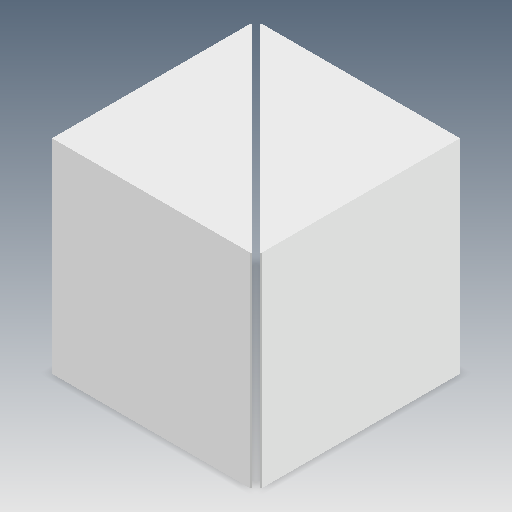
# Autodesk Inventor part: Beamsplittertransparent
Saved by Autodesk Inventor 2026 (Build 300175050, 175E)
## iProperties
Created: 2025-08-02
Part Number: Beamsplittertransparent
Material: Generic
Document SubType Name: Modeling
Designer: aman0
Density: 1 g/cm^3
Appearance: Default
Author: aman0
Autodesk Inventor part; units mm, degrees
ref_plane "YZ Plane" through (0, 0, 0) normal (1, 0, 0) x (0, 1, 0)
ref_plane "XZ Plane" through (0, 0, 0) normal (0, 1, 0) x (-1, 0, 0)
ref_plane "XY Plane" through (0, 0, 0) normal (0, 0, 1) x (1, 0, 0)
sketch "Sketch1" plane through (0, 0, 0) normal (0, 1, 0) x (-1, 0, 0)
  line L0 (-12.5, 12) -> (-12.5, -12.5)
  line L1 (-12.5, -12.5) -> (12, -12.5)
  line L2 (12.5, -12) -> (12.5, 12.5)
  line L3 (12.5, 12.5) -> (-12, 12.5)
  line L4 (-12.5, 12.5) -> (12.5, -12.5) construction
  line L5 (-12.5, -12.5) -> (12.5, 12.5) construction
  line L6 (12, -12.5) -> (-12.5, 12)
  line L7 (12.5, -12) -> (-12, 12.5)
  point P0 (0, 0)
  point P1 (0, 0)
  point P2 (0, 0)
  dimension "d13" = 1
  dimension "d14" = 2
  dimension "d15" = 0.3535
  dimension "d0" = 25
  dimension "d1" = 25
  dimension "d2" = 0.5
  dimension "d3" = 0.5
  dimension "d4" = 0.5
  dimension "d5" = 0.7071
  dimension "d6" = 17.6777
  dimension "d7" = 17.6777
  dimension "d8" = 24.5
  constraints: 16 end point, 4 midpoint, 3 parallel, 1 perpendicular, 1 vertical
  measures "d0" distance of L4.start L0.end
  measures "d1" distance of L4.end L0.end
  measures "d2" distance of L1.end L4.end
  measures "d3" distance of L0.start L4.start
  measures "d4" distance of L3.end L4.start
  measures "d5" distance between parallel lines of L6 L7
  measures "d6" distance of point (0, 0) L2.end
  measures "d7" distance of point (0, 0) L0.end
  measures "d8" distance of L2.start L2.end
extrude "Extrusion1" add sketch "Sketch1" along normal mid plane 25
sketch "Sketch3" plane through (0, 12.5, 0) normal (0, 1, 0) x (1, 0, 0)
  line L0 (-13.9142, 13.2071) -> (-13.2071, 13.9142)
  line L1 (-13.2071, 13.9142) -> (-11.7929, 12.5)
  line L2 (-11.7929, 12.5) -> (-12.5, 11.7929)
  line L3 (-12.5, 11.7929) -> (-13.9142, 13.2071)
  line L4 (-13.9142, 13.2071) -> (-11.7929, 12.5) construction
  line L5 (-13.2071, 13.9142) -> (-12.5, 11.7929) construction
  line L6 (12, -12.5) -> (-12.5, 12) projected
  line L7 (-12.5, 12) -> (-12.5, -12.5) projected
  line L8 (13.2071, -13.9142) -> (13.9142, -13.2071)
  line L9 (13.9142, -13.2071) -> (12.5, -11.7929)
  line L10 (12.5, -11.7929) -> (11.7929, -12.5)
  line L11 (11.7929, -12.5) -> (13.2071, -13.9142)
  line L12 (13.2071, -13.9142) -> (12.5, -11.7929) construction
  line L13 (13.9142, -13.2071) -> (11.7929, -12.5) construction
  line L14 (-12, 12.5) -> (12.5, -12) projected
  line L15 (-12.5, -12.5) -> (12, -12.5) projected
  line L16 (12.5, -12) -> (12.5, 12.5) projected
  point P0 (0, 0)
  point P1 (-12.8536, 12.8536)
  point P2 (-12.8536, 12.8536)
  point P3 (12.8536, -12.8536)
  point P4 (12.8536, -12.8536)
  dimension "d13" = 1
  dimension "d14" = 2
  dimension "d15" = 0.3535
  dimension "d16" = 1
  dimension "d17" = 0.3535
  dimension "d18" = 2
  constraints: 24 end point, 6 midpoint, 4 parallel, 3 point on line, 2 perpendicular
  measures "d13" distance of L0.start L0.end
  measures "d14" distance of L0.end L1.end
  measures "d15" distance from line of point (-12.854, 12.854) L6
  measures "d16" distance of L8.start L8.end
  measures "d17" distance from line of L14 point (12.854, -12.854)
  measures "d18" distance of L8.end L9.end
extrude "Extrusion3" cut sketch "Sketch3" against normal through all contours L0 L1 L2 L6 L7 L3 | L7 L6 L2 | L10 L14 L16 L9 L8 L11 L15 L6 | L6 L15 L10 | L10 L16 L14
body "Solid1"
